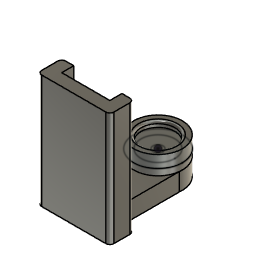
End piece v11 v6 (Autodesk Fusion 360 design; units mm, degrees)
Autodesk Fusion 360 part; units mm, degrees
sketch "Sketch1" plane through (0, 0, 0) normal (0, 0, 1) x (1, 0, 0)
  circle A0 centre (0, 0) radius 15.1
  circle A1 centre (0, 0) radius 10.55
  circle A2 centre (0, 0) radius 3.05
  dimension "d1" = 30.2
  dimension "d2" = 21.1
  dimension "d3" = 6.1
  constraint coincident A0.centre A1.centre
  constraint concentric A0 A1
  constraint concentric A1 A2
  measures "d1" diameter of A0
  measures "d2" diameter of A1
  measures "d3" diameter of A2
extrude "Extrude1" add sketch "Sketch1" along normal blind 7.5 contours A0 makes body 1
extrude "Extrude2" add sketch "Sketch1" along normal blind 3 contours A1 | A2 bodies 1
extrude "Extrude3" cut sketch "Sketch1" along normal blind 4 contours A2 bodies 1
extrude "Extrude4" add 1 faces at (8.0107, -0.5241, 3) along direction (0, 0, 1) blind 1 on bodies 1 bodies 1
extrude "Extrude5" add 1 faces at (11.0158, -0.9017, 0) along direction (0, 0, -1) blind 2 on bodies 1 bodies 1
extrude "Extrude6" add sketch "Sketch1" along normal blind 4 and the other way blind -2 contours A2 bodies 1
extrude "Extrude7" add 1 faces at (11.0158, -0.9017, -2) along direction (0, 0, -1) blind 12 and the other way blind -4 on bodies 1 bodies 1 makes body 2
extrude "Extrude8" add 1 faces at (11.0158, -0.9017, -2) along direction (0, 0, -1) blind 2 on bodies 1 bodies 1
sketch "Sketch2" plane through (0, 0, 0) normal (0, 1, 0) x (1, 0, 0)
extrude "Extrude9" add 1 faces at (11.0158, -0.9017, -14) along direction (0, 0, -1) blind 3 on bodies 2 bodies 2
sketch "Sketch3" plane through (0, 0, 0) normal (0, 1, 0) x (1, 0, 0)
  line L0 (-15, 17) -> (15, 17)
  line L1 (15, 17) -> (15, 6)
  line L2 (15, 6) -> (-15, 6)
  line L3 (-15, 6) -> (-15, 17)
  constraint horizontal L0
  constraint vertical L1
  constraint horizontal L2
  constraint vertical L3
extrude "Extrude10" add sketch "Sketch3" against normal blind 50 bodies 2
extrude "Extrude11" cut sketch "Sketch1" against normal blind 23 contours A2 bodies 2
extrude "Extrude12" cut 1 faces at (-5, -50, -13.3333) along direction (0, 1, 0) blind 5 on bodies 2 bodies 2
sketch "Sketch4" plane through (0, 0, -6) normal (0, 0, 1) x (-1, 0, 0)
  circle A0 centre (0, 0) radius 3.05
  arc A1 (-15, 1.7349) -> (15, 1.7349) centre (0, 0) ccw
  line L0 (15, 1.7349) -> (15, 45)
  line L1 (15, 45) -> (-15, 45)
  line L2 (-15, 45) -> (-15, 1.7349)
  line L3 (22.5, 37.5) -> (-22.5, 37.5)
  line L4 (-22.5, 37.5) -> (-22.5, 52.5)
  line L5 (-22.5, 52.5) -> (22.5, 52.5)
  line L6 (22.5, 52.5) -> (22.5, 37.5)
  line L7 (22.5, 37.5) -> (-22.5, 52.5) construction
  line L8 (-22.5, 37.5) -> (22.5, 52.5) construction
  point P0 (0, 45)
  dimension "d36" = 15
  constraint horizontal L3
  constraint perpendicular L3 L4
  constraint parallel L3 L5
  constraint parallel L4 L6
  constraint coincident L7 P0
  constraint coincident L8 P0
  constraint midpoint L1 P0
  measures "d36" distance of L3 L5
extrude "Extrude13" add sketch "Sketch4" along normal blind 55 and the other way blind 11 contours L0 L1 L2 L3 L4 L5 L6 bodies 2
extrude "Extrude14" add 1 faces at (5, -50, 49) along direction (0, 0, 1) blind 10 on bodies 2 bodies 2
extrude "Extrude15" cut 1 faces at (5, -50, 59) along direction (0, 0, -1) blind 10 on bodies 2 bodies 2
extrude "Extrude16" add 1 faces at (5, -50, 49) along direction (0, 0, 1) blind 5 on bodies 2 bodies 2
extrude "Extrude17" add 1 faces at (5, -50, 54) along direction (0, 0, 1) blind 0.325 on bodies 2 bodies 2
extrude "Extrude18" cut 1 faces at (5, -50, 54.325) along direction (0, 0, -1) blind 0.325 on bodies 2 bodies 2
fillet "Fillet1" radius 2.5 4 edges at (22.5, -52.5, 18.5) (22.5, -37.5, 18.5) (-22.5, -37.5, 18.5) (-22.5, -52.5, 18.5) on bodies 2
move_body "Move1" bodies 2 to x (1, 0, 0) y (0, 1, 0) z (0, 0, 1) at (0, 0, 2)
fillet "Fillet2" radius 1.5 1 edges at (-9.8361, 3.815, 7.5) on bodies 1
